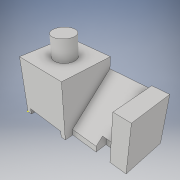
# Autodesk Inventor part: 400185627_VD
Saved by Autodesk Inventor 2017 (Build 210142000, 142)
## iProperties
Created: 2019-01-15
Part Number: 400185627_VD
Material: Generic
Document SubType Name: Modeling
Designer: STUDENT21
Density: 1 g/cm^3
Appearance: Default
Author: STUDENT21
Autodesk Inventor part; units mm, degrees
ref_plane "YZ Plane" through (0, 0, 0) normal (1, 0, 0) x (0, 1, 0)
ref_plane "XZ Plane" through (0, 0, 0) normal (0, 1, 0) x (-1, 0, 0)
ref_plane "XY Plane" through (0, 0, 0) normal (0, 0, 1) x (1, 0, 0)
sketch "Sketch1" plane through (0, 0, 0) normal (0, 1, 0) x (-1, 0, 0)
  line L0 (0, 0) -> (-50, 0)
  line L1 (-50, 0) -> (-50, -50)
  line L2 (-50, -50) -> (0, -50)
  line L3 (0, -50) -> (0, 0)
  dimension "d0" = 50
  dimension "d1" = 50
  constraints: 8 end point, 2 parallel, 1 horizontal, 1 perpendicular
  measures "d0" distance of L2.end L1.end
  measures "d1" distance of L1.end L0.end
extrude "Extrusion1" add sketch "Sketch1" along normal blind 55
sketch "Sketch2" plane through (0, 0, 0) normal (0, 0, 1) x (1, 0, 0)
  line L0 (0, 0) -> (50, 0) projected
  line L1 (45, 0) -> (45, 6)
  line L2 (50, 0) -> (50, 55) projected
  line L3 (5, 0) -> (5, 6)
  line L4 (0, 0) -> (0, 55) projected
  line L5 (5, 6) -> (45, 6)
  line L6 (5, 0) -> (45, 0)
  dimension "d7" = 6
  dimension "d8" = 5
  dimension "d9" = 5
  constraints: 8 end point, 2 perpendicular, 2 point on line, 1 collinear, 1 vertical
  measures "d7" distance of L1.start L1.end
  measures "d8" distance between parallel lines of L2 L1
  measures "d9" distance between parallel lines of L4 L3
sketch "Sketch3" plane through (0, 0, 0) normal (0, 0, 1) x (1, 0, 0)
  point P0 (0, 0)
sketch "Sketch4" plane through (0, 55, 0) normal (0, 1, 0) x (1, 0, 0)
  circle A0 centre (25, 25) radius 10.5
  line L0 (0, 50) -> (0, 0) projected
  line L1 (0, 0) -> (50, 0) projected
  dimension "d10" = 21
  dimension "d11" = 25
  dimension "d12" = 25
  constraints: 1 centre point
  measures "d10" diameter of A0
  measures "d11" distance from line of L0 A0.centre
  measures "d12" distance from line of L1 A0.centre
extrude "Extrusion2" cut sketch "Sketch2" against normal blind 55
extrude "Extrusion3" add sketch "Sketch4" along normal blind 20
sketch "Sketch5" plane through (50, 0, 0) normal (1, 0, 0) x (0, 0, -1)
  line L0 (50, 0) -> (8, 0)
  line L1 (0, 0) -> (50, 0) projected
  line L2 (8, 0) -> (8, 6)
  line L3 (0, 55) -> (50, 55) projected
  line L4 (50, 0) -> (50, 55) projected
  line L5 (50, 0) -> (50, 44)
  line L6 (8, 6) -> (50, 44)
  dimension "d17" = 42
  dimension "d18" = 6
  dimension "d27" = 44
  constraints: 8 end point, 2 point on line, 1 vertical
  measures "d17" distance of L0.start L0.end
  measures "d18" distance of L0.end L2.end
  measures "d27" distance of L0.start L5.end
extrude "Extrusion4" add sketch "Sketch5" along normal blind 40
sketch "Sketch6" plane through (50, 0, -8) normal (0, 0, 1) x (1, 0, 0)
  point P0 (-50, 0)
sketch "Sketch7" plane through (50, 6, -8) normal (0, 0.6987, 0.7154) x (1, 0, 0)
  point P0 (-50, -9.8822)
sketch "Sketch8" plane through (50, 6, -8) normal (0, 0.6987, 0.7154) x (1, 0, 0)
  point P0 (-50, -9.8822)
sketch "Sketch9" plane through (90, 0, 0) normal (1, 0, 0) x (0, 0, -1)
  line L0 (0, 0) -> (50, 0) projected
  line L1 (50, 0) -> (8, 0)
  line L2 (8, 0) -> (8, 47)
  line L3 (8, 47) -> (50, 47)
  line L4 (50, 47) -> (50, 0)
  dimension "d22" = 42
  dimension "d23" = 47
  constraints: 8 end point, 2 parallel, 1 horizontal, 1 perpendicular
  measures "d22" distance of L2.end L3.end
  measures "d23" distance of L1.end L2.end
extrude "Extrusion5" add sketch "Sketch9" along normal blind 15
sketch "Sketch10" plane through (50, 0, -8) normal (0, 0, 1) x (1, 0, 0)
  point P0 (-50, 0)
sketch "Sketch11" plane through (50, 0, -8) normal (0, 0, 1) x (1, 0, 0)
  line L0 (40, 0) -> (26, 0)
  line L1 (26, 0) -> (26, 12)
  line L2 (26, 12) -> (40, 12)
  line L3 (40, 12) -> (40, 0)
  point P0 (-50, 0)
  dimension "d28" = 14
  dimension "d29" = 12
  constraints: 8 end point, 2 parallel, 1 horizontal, 1 perpendicular
  measures "d28" distance of L1.end L2.end
  measures "d29" distance of L0.end L1.end
extrude "Extrusion6" cut sketch "Sketch11" against normal blind 11
body "Solid1"
